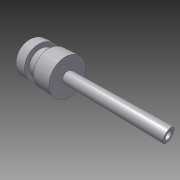
# Autodesk Inventor part: hotend_mount
Saved by Autodesk Inventor 2014 (Build 180170000, 170)
## iProperties
Created: 2014-03-25
Part Number: hotend_mount
Material: Aluminum 6061
Document SubType Name: Modeling
Designer: buben
Density: 2.71 g/cm^3
Appearance: Aluminum - Flat
Mass: 9.53813 g
Surface Area: 25.268 cm^2
Volume: 3.5196 cm^3
Author: buben
Autodesk Inventor part; units mm, degrees
ref_plane "YZ Plane" through (0, 0, 0) normal (1, 0, 0) x (0, 1, 0)
ref_plane "XZ Plane" through (0, 0, 0) normal (0, 1, 0) x (-1, 0, 0)
ref_plane "XY Plane" through (0, 0, 0) normal (0, 0, 1) x (1, 0, 0)
sketch "Sketch1" plane through (0, 0, 0) normal (0, 0, 1) x (1, 0, 0)
  line L0 (0, 0) -> (0, 8)
  line L1 (0, 8) -> (5, 8)
  line L2 (5, 8) -> (5, 6)
  line L3 (5, 6) -> (10, 6)
  line L4 (10, 6) -> (10, 8)
  line L5 (10, 8) -> (18, 8)
  line L6 (18, 8) -> (18, 0)
  line L7 (18, 0) -> (0, 0)
  dimension "d0" = 18
  dimension "d1" = 5
  dimension "d2" = 5
  dimension "d3" = 2
  dimension "d4" = 8
  constraints: 16 end point, 5 parallel, 2 collinear, 1 perpendicular, 1 vertical
  measures "d0" distance of L6.end L0.start
  measures "d1" distance of L0.end L1.end
  measures "d2" distance of L2.end L3.end
  measures "d3" distance of L1.end L2.end
  measures "d4" distance of L5.end L6.end
revolve "Revolution1" add sketch "Sketch1" angle 360 about axis through (18, 0, 0) along (-1, 0, 0)
sketch "Sketch2" plane through (0, 0, 0) normal (-1, 0, 0) x (0, 0, 1)
  circle A0 centre (0, 0) radius 8 projected
hole "Hole1" at (0, 0, 0) direction (1, 0, 0) diameter 3 end through all countersink diameter 5 countersink angle 60
sketch "Sketch3" plane through (18, 0, 0) normal (1, 0, 0) x (0, 0, -1)
  circle A0 centre (0, 0) radius 1.5 projected
  circle A1 centre (0, 0) radius 8 projected
  circle A2 centre (0, 0) radius 2.5
  dimension "d13" = 5
  constraints: 1 centre point, 1 coincident
  measures "d13" diameter of A2
extrude "Extrusion1" add sketch "Sketch3" along normal blind 38 contours A2
body "Solid1"
